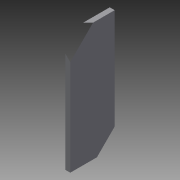
# Autodesk Inventor part: Yagi_BaseFrame
Saved by Autodesk Inventor 2014 (Build 180170000, 170)
## iProperties
Created: 2015-01-07
Part Number: Yagi_BaseFrame
Material: Generic
Document SubType Name: Modeling
Designer: Owner
Density: 1 g/cm^3
Appearance: Default
Author: Owner
Autodesk Inventor part; units mm, degrees
ref_plane "YZ Plane" through (0, 0, 0) normal (1, 0, 0) x (0, 1, 0)
ref_plane "XZ Plane" through (0, 0, 0) normal (0, 1, 0) x (-1, 0, 0)
ref_plane "XY Plane" through (0, 0, 0) normal (0, 0, 1) x (1, 0, 0)
sketch "Sketch1" plane through (0, 0, 0) normal (0, 0, 1) x (1, 0, 0)
  line L0 (65.2483, 137.2649) -> (65.2483, -15.1351)
  line L1 (71.5983, 137.2649) -> (71.5983, -15.1351)
  line L2 (65.2483, -15.1351) -> (71.5983, -15.1351)
  line L3 (65.2483, 137.2649) -> (71.5983, 137.2649)
  line L4 (65.2483, 128.3749) -> (65.2483, 131.5499)
  line L5 (65.2483, 47.6029) -> (65.2483, 44.4279)
  point P0 (0, 0)
  dimension "d1" = 152.4
  dimension "d21" = 6.35
  constraints: 12 end point, 2 point on line, 1 horizontal, 1 parallel, 1 perpendicular
  measures "d1" distance of L0.start L0.end
  measures "d21" distance of L0.start L1.start
extrude "Extrusion1" add sketch "Sketch1" along normal blind 57.15
body "Solid1"
